nixal_reprap_ZbracketCompatible_non4040 (Autodesk Fusion 360 design; units mm, degrees)
Autodesk Fusion 360 part; units mm, degrees
sketch "Sketch1" plane through (0, 0, 0) normal (0, 1, 0) x (1, 0, 0)
  circle A0 centre (0, 0) radius 4
  circle A1 centre (21, -2) radius 4
  line L0 (-8, 31) -> (41, 31)
  line L1 (41, 31) -> (41, -3)
  line L2 (30, -14) -> (2, -14)
  line L3 (-0.0855, 23) -> (41, 23)
  circle A2 centre (21, -2) radius 4
  line L4 (25.1, 31) -> (16.9, 31)
  line L5 (16.9, 31) -> (16.9, 35.4)
  line L6 (16.9, 35.4) -> (25.1, 35.4)
  line L7 (25.1, 35.4) -> (25.1, 31)
  line L8 (25.1, 31) -> (16.9, 35.4) construction
  line L9 (16.9, 31) -> (25.1, 35.4) construction
  line L10 (36.5, 13.5) -> (5.5, 13.5) construction
  line L11 (-0.0855, 31) -> (-0.0855, 14.4309)
  arc A3 (30, -14) -> (41, -3) centre (30, -3) ccw
  line L12 (-0.0855, 15.3033) -> (-0.0855, 11)
  line L13 (-12.2341, -5.0001) -> (-12.2341, 5)
  line L14 (-9.2341, 8) -> (-3.0868, 8)
  line L15 (-0.088, 11.0855) -> (-0.0855, 11)
  line L16 (-9.2341, -8.0001) -> (-3.0855, -8.0001)
  line L17 (-0.0855, -11.0001) -> (-0.0855, -11)
  line L18 (2.9145, -14) -> (2.7644, -14)
  line L19 (-12.2341, -1.5) -> (-3.7081, -1.5)
  line L20 (-12.2341, 1.5) -> (-3.7081, 1.5)
  arc A4 (-9.2341, 8) -> (-12.2341, 5) centre (-9.2341, 5) ccw
  arc A5 (-12.2341, -5.0001) -> (-9.2341, -8.0001) centre (-9.2341, -5.0001) ccw
  arc A6 (-3.0868, 8) -> (-0.088, 11.0855) centre (-3.0868, 11) ccw
  arc A7 (-0.0855, -11.0001) -> (-3.0855, -8.0001) centre (-3.0855, -11.0001) ccw
  arc A8 (-0.0855, -11) -> (2.9145, -14) centre (2.9145, -11) ccw
  dimension "d1" = 8
  dimension "d2" = 8
  dimension "d4" = 49
  dimension "d6" = 31
  dimension "d9" = 8
  dimension "d18" = 20
  dimension "d19" = 33
  dimension "d23" = 8
  dimension "d43" = 20
  dimension "d44" = 2.2
  dimension "d45" = 4.4
  dimension "d46" = 8.2
  dimension "d67" = 41
  dimension "d82" = 1.5
  dimension "d83" = 8.526
  dimension "d84" = 1.5
  dimension "d85" = 3
  dimension "d86" = 3
  dimension "d87" = 3
  dimension "d88" = 3
  dimension "d89" = 3
  constraint coincident A0.centre origin
  constraint horizontal L0
  constraint vertical L1
  constraint coincident L1
  constraint perpendicular L1 L3
  constraint concentric A1 A2
  constraint perpendicular L4 L5
  constraint parallel L4 L6
  constraint parallel L5 L7
  constraint horizontal L4
  constraint coincident L8 A0.centre
  constraint coincident L9 A0.centre
  constraint horizontal L10
  constraint vertical L11
  constraint tangent L1 A3
  constraint tangent L2 A3
  constraint coincident L11
  constraint parallel L11 L12
  constraint vertical L13
  constraint perpendicular L13 L16
  constraint coincident L13 A0.centre
  constraint coincident A0 origin
  constraint perpendicular L13 L19
  constraint perpendicular L13 L20
  constraint tangent L14 A4
  constraint tangent L13 A4
  constraint tangent L13 A5
  constraint tangent L16 A5
  constraint tangent L14 A6
  constraint tangent L15 A6
  constraint tangent L16 A7
  constraint tangent L18 A8
  measures "d1" diameter of A0
  measures "d2" diameter of A1
  measures "d6" distance of A0.centre L0
  measures "d9" distance of L0 L3
  measures "d18" distance of A0.centre L1
  measures "d19" distance of A0.centre L0
  measures "d23" diameter of A2
  measures "d43" distance of A0.centre
  measures "d44" distance of L0 A0.centre
  measures "d67" distance of A0.centre L1
  measures "d85" radius of A4
  measures "d86" radius of A5
  measures "d87" radius of A6
  measures "d88" radius of A7
  measures "d89" radius of A8
extrude "Extrude1" add sketch "Sketch1" along normal blind 9 contours A0 L1 L2 L3 L11 A3 L12 L13 L14 L15 L16 L19 L20 A4 A5 A6 A7 A8 | L0 L1 L3 L4 L11 | A1 A2
extrude "Extrude2" add sketch "Sketch1" along normal blind 22.5 and the other way blind -8 contours L0 L1 L3 L4 L11
sketch "Sketch2" plane through (0, 0, -23) normal (0, 0, 1) x (1, 0, 0)
  line L0 (-0.0855, 9) -> (41, 9)
  line L1 (41, 9) -> (41, 22.5)
  line L2 (41, 22.5) -> (-0.0855, 22.5)
  circle A0 centre (31, 9.5) radius 1.65
  circle A1 centre (11, 9.5) radius 1.65
  circle A2 centre (11, 9.5) radius 2.75
  circle A3 centre (31, 9.5) radius 2.7
  circle A4 centre (21, 13.5) radius 4
  circle A5 centre (21, 13.5) radius 7.5
  line L3 (-0.0855, 22.5) -> (-0.0855, 9)
  line L4 (2.9212, 22.5005) -> (38, 22.5005)
  line L5 (41, 19.5005) -> (41, 9)
  line L6 (41, 9) -> (-0.0788, 9)
  line L7 (-0.0788, 9) -> (-0.0788, 19.5005)
  arc A6 (2.9212, 22.5005) -> (-0.0788, 19.5005) centre (2.9212, 19.5005) ccw
  arc A7 (41, 19.5005) -> (38, 22.5005) centre (38, 19.5005) ccw
  dimension "d13" = 3.3
  dimension "d14" = 3.3
  dimension "d15" = 20
  dimension "d20" = 10
  dimension "d21" = 13
  dimension "d22" = 13
  dimension "d27" = 5.5
  dimension "d28" = 5.4
  dimension "d31" = 8
  dimension "d32" = 20
  dimension "d33" = 9
  dimension "d36" = 15
  dimension "d74" = 3
  dimension "d75" = 3
  constraint concentric A1 A2
  constraint concentric A0 A3
  constraint concentric A4 A5
  constraint horizontal L4
  constraint vertical L5
  constraint horizontal L6
  constraint vertical L7
  constraint tangent L7 A6
  constraint tangent L4 A6
  constraint tangent L4 A7
  constraint tangent L5 A7
  measures "d13" diameter of A0
  measures "d14" diameter of A1
  measures "d20" distance of L1
  measures "d27" diameter of A2
  measures "d28" diameter of A3
  measures "d31" diameter of A4
  measures "d32" distance of L1 origin
  measures "d36" diameter of A5
  measures "d74" radius of A6
  measures "d75" radius of A7
extrude "Extrude3" cut sketch "Sketch2" against normal blind 18 contours L0 A1 L6 | L0 A1 L6 | L0 A0 L6 | L0 A0 L6
extrude "Extrude4" cut sketch "Sketch1" along normal blind 14 and the other way blind 13 contours A0 | A1 A2
extrude "Extrude5" cut sketch "Sketch2" against normal blind 2 contours L0 A1 A2 L6 | L0 A1 A2 L6 | L0 A0 A3 L6 | L0 A0 A3 L6
sketch "Sketch3" plane through (0, 0, 8.0001) normal (0, 0, 1) x (1, 0, 0)
  line L0 (-9.2341, 0) -> (-3.0855, 0)
  line L1 (-3.0855, 9) -> (-9.2341, 9)
  line L2 (-9.2341, 9) -> (-3.0855, 9)
  line L3 (-3.0855, 9) -> (-3.0855, 0)
  line L4 (-3.0855, 0) -> (-9.2341, 0)
  line L5 (-9.2341, 0) -> (-9.2341, 9)
  circle A0 centre (-6.1598, 4.5) radius 1.6
  line L6 (-9.2341, 9) -> (-9.2341, 0)
  line L7 (-3.0855, 0) -> (-3.0855, 9)
  line L8 (-9.2341, 9) -> (-3.0855, 0) construction
  line L9 (-3.0855, 9) -> (-9.2341, 0) construction
  dimension "d79" = 3.2
  constraint horizontal L2
  constraint vertical L3
  constraint horizontal L4
  constraint vertical L5
  constraint midpoint L9
  measures "d79" diameter of A0
extrude "Extrude12" cut sketch "Sketch3" against normal blind 23 contours A0
extrude "Extrude13" cut sketch "Sketch2" against normal blind 24 contours L0 L2 L3 L7 A6 | L1 L2 A7
extrude "Extrude14" cut sketch "Sketch2" along normal blind 42 contours L0 A1 A2 L6 | L0 A1 L6 | L0 A0 A3 L6 | L0 A0 L6 picked at (13.293, 8.8705) picked at (10.8308, 8.5784) picked at (28.7406, 8.8733) picked at (30.9896, 8.5424)
extrude "Extrude15" add sketch "Sketch1" along normal blind 22.5 contours L0 L4 L5 L6 L7
extrude "Extrude16" cut sketch "Sketch2" against normal blind 39 contours A4
